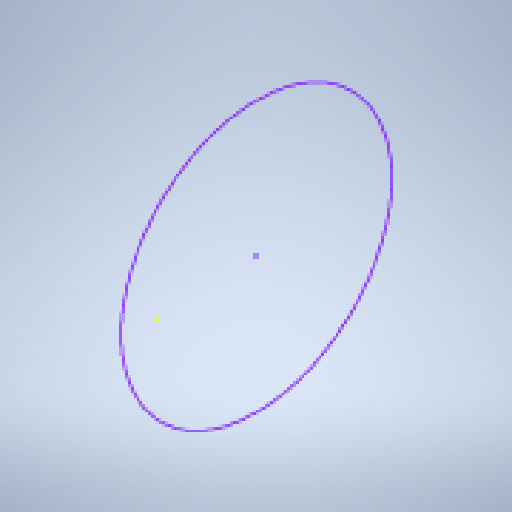
# Autodesk Inventor part: PulleyMover
Saved by Autodesk Inventor 2023 (Build 270158000, 158)
## iProperties
Created: 2022-09-25
Part Number: PulleyMover
Material: Generic
Document SubType Name: Modeling
Designer: deli
Density: 1 g/cm^3
Appearance: Default
Author: deli
Autodesk Inventor part; units mm, degrees
ref_plane "YZ Plane" through (0, 0, 0) normal (1, 0, 0) x (0, 1, 0)
ref_plane "XZ Plane" through (0, 0, 0) normal (0, 1, 0) x (-1, 0, 0)
ref_plane "XY Plane" through (0, 0, 0) normal (0, 0, 1) x (1, 0, 0)
sketch "Sketch1" plane through (0, 0, 0) normal (1, 0, 0) x (0, 1, 0)
  circle A0 centre (32.8182, 3.5633) radius 7
  circle A1 centre (32.7593, -52.7466) radius 7
  arc A2 (27.7506, -47.8566) -> (27.7993, -1.3162) centre (3.89, -24.5614) ccw
  arc A3 (37.7681, -57.6366) -> (37.8372, 8.4429) centre (3.89, -24.5614) ccw
  line L0 (22.2002, 6.4368) -> (6.2609, -52.4609)
  line L1 (6.2609, -52.4609) -> (28.0857, -62.7043)
  arc A4 (40.6302, -60.4309) -> (40.7052, 11.2312) centre (3.89, -24.5614) ccw
  arc A5 (40.7052, 11.2312) -> (22.2002, 6.4368) centre (32.8182, 3.5633) ccw
  arc A6 (28.0857, -62.7043) -> (40.6302, -60.4309) centre (32.7593, -52.7466) ccw
  circle A7 centre (6.2609, -52.4609) radius 55
  circle A8 centre (6.2609, -52.4609) radius 69
  point P0 (0, 0)
  dimension "d1" = 14
  dimension "d3" = 14
  dimension "d5" = 26.5
  dimension "d7" = 14
  dimension "d8" = 28
  dimension "d9" = 4
  dimension "d10" = 4
  dimension "d11" = 100
  dimension "d12" = 62
  dimension "d13" = 4
  constraints: 14 point on circle, 9 centre point, 6 coincident, 6 tangent, 4 end point
  measures "d1" diameter of A0
  measures "d3" diameter of A1
  measures "d5" distance of L0.end A1.centre
  measures "d7" radial gap between concentric circles of A2 A3
  measures "d8" distance of L0.end A2.centre
  measures "d9" distance edge to line of A1 L1
  measures "d10" distance edge to line of A0 L0
  measures "d11" angle of L1 L0
  measures "d12" distance of A0.centre L0.end
  measures "d13" radial gap between concentric circles of A3 A4
extrude "Extrusion1" add sketch "Sketch1" along normal blind 3.175 contours A0 A8 A4 A7 A3 | A8 A5 A4 | A0 A2 A7 L0 A5 A8 | A7 A4 A6 L1 L0 A2 A1 A3
equation "\"d3\" = d1"
body "Solid1"
